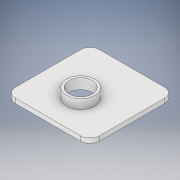
# Autodesk Inventor part: case_top
Saved by Autodesk Inventor 2019 (Build 230136000, 136)
## iProperties
Created: 2019-01-23
Part Number: case_top
Material: Generic
Document SubType Name: Modeling
Designer: jmc
Density: 1 g/cm^3
Appearance: PET White
Author: jmc
Autodesk Inventor part; units mm, degrees
ref_plane "YZ Plane" through (0, 0, 0) normal (1, 0, 0) x (0, 1, 0)
ref_plane "XZ Plane" through (0, 0, 0) normal (0, 1, 0) x (-1, 0, 0)
ref_plane "XY Plane" through (0, 0, 0) normal (0, 0, 1) x (1, 0, 0)
sketch "Sketch2" plane through (0, 0, 0) normal (0, 1, 0) x (-1, 0, 0)
  line L0 (90, 70) -> (90, -70)
  arc A0 (70, -90) -> (90, -70) centre (70, -70) ccw
  line L1 (70, -90) -> (-70, -90)
  arc A1 (-90, -70) -> (-70, -90) centre (-70, -70) ccw
  line L2 (-90, -70) -> (-90, 70)
  arc A2 (-70, 90) -> (-90, 70) centre (-70, 70) ccw
  line L3 (-70, 90) -> (70, 90)
  arc A3 (90, 70) -> (70, 90) centre (70, 70) ccw
  line L4 (-90, 90) -> (90, -90)
  line L5 (90, 90) -> (-90, -90)
  line L6 (0, 101.9126) -> (0, -124.7005)
  line L7 (136.9186, 0) -> (-105.9116, 0)
  point P0 (0, 0)
  constraints: 16 end point, 8 point on circle, 8 tangent, 4 centre point, 4 perpendicular, 3 equal radius, 2 parallel
extrude "Extrusion1" add sketch "Sketch2" along normal blind 10
shell "Shell1" thickness 2 removed faces 1 at (23.3333, 0, 30)
sketch "Sketch3" plane through (0, 10, 0) normal (0, 1, 0) x (1, 0, 0)
  circle A0 centre (0, -20) radius 25.075
  line L0 (70, 90) -> (-70, 90) projected
  point P0 (0, 0)
  dimension "d6" = 50.15
  dimension "d7" = 0
  dimension "d8" = 110
  constraints: 1 centre point
  measures "d6" diameter of A0
  measures "d7" horizontal distance of point (0, 0) A0.centre
  measures "d8" distance from line of A0.centre L0
extrude "agujero del comedero" cut sketch "Sketch3" against normal blind 10
sketch "Sketch4" plane through (0, 10, 0) normal (0, 1, 0) x (1, 0, 0)
  circle A0 centre (0, -20) radius 25.075 projected
  circle A1 centre (0, -20) radius 30.075
  point P0 (0, 0)
  dimension "d11" = 5
  constraints: 1 centre point
  measures "d11" radial gap between concentric circles of A0 A1
extrude "Extrusion3" add sketch "Sketch4" along normal blind 20
body "Solid1"
